# Autodesk Inventor part: 4_7K
Saved by Autodesk Inventor 2016 (Build 200138000, 138)
## iProperties
Created: 2016-04-08
Part Number: 4_7K
Material: Generic
Document SubType Name: Modeling
Designer: Paschalis
Density: 1 g/cm^3
Appearance: R3216, 4_7K
Author: Paschalis
Autodesk Inventor part; units mm, degrees
ref_plane "YZ Plane" through (0, 0, 0) normal (1, 0, 0) x (0, 1, 0)
ref_plane "XZ Plane" through (0, 0, 0) normal (0, 1, 0) x (-1, 0, 0)
ref_plane "XY Plane" through (0, 0, 0) normal (0, 0, 1) x (1, 0, 0)
sketch "R3216, 4_7K_91" plane through (0, 0, 0) normal (0, 0, 1) x (1, 0, 0)
  line L0 (-2.473, 0.983) -> (2.473, 0.983)
  line L1 (2.473, 0.983) -> (2.473, -0.983)
  line L2 (2.473, -0.983) -> (-2.473, -0.983)
  line L3 (-2.473, -0.983) -> (-2.473, 0.983)
  constraints: 8 end point
extrude "Extrusion1" add sketch "R3216, 4_7K_91" along normal blind 1
body "Solid1"
